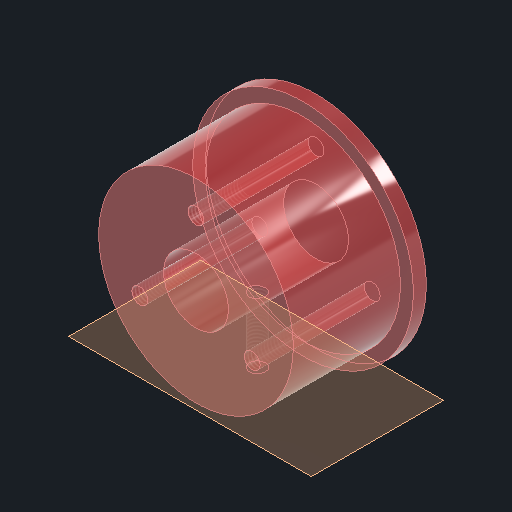
# Autodesk Inventor part: ReelMotorBearingShaft
Saved by Autodesk Inventor 2027 (Build 310192060, 192F)
## iProperties
Created: 2024-02-11
Part Number: ReelMotorBearingShaft
Material: Aluminum 6061
Document SubType Name: Modeling
Designer: Vinicius
Density: 2.7 g/cm^3
Appearance: Dark Red
Mass: 31.7586 g
Surface Area: 44.0893 cm^2
Volume: 11.7624 cm^3
Author: Vinicius
Autodesk Inventor part; units mm, degrees
ref_plane "YZ Plane" through (0, 0, 0) normal (1, 0, 0) x (0, 1, 0)
ref_plane "XY Plane" through (0, 0, 0) normal (0, 0, 1) x (1, 0, 0)
sketch "Sketch1" plane through (0, 0, 0) normal (0, 1, 0) x (-1, 0, 0)
  line L0 (0, 0) -> (0, 34.0434)
  line L1 (5, 0) -> (5, 18.5)
  line L2 (5, 18.5) -> (15, 18.5)
  line L3 (15, 18.5) -> (15, 2)
  line L4 (15, 2) -> (17, 2)
  line L5 (17, 2) -> (17, 0)
  line L6 (17, 0) -> (5, 0)
  dimension "d0" = 10
  dimension "d1" = 2
  dimension "d2" = 2
  dimension "d3" = 30
  dimension "d4" = 16.5
  constraints: 14 end point, 5 perpendicular, 2 vertical, 1 horizontal alignment
  measures "d0" diameter of L1 L0
  measures "d1" distance from line of L4.end L3
  measures "d2" distance of L4.end L5.end
  measures "d3" diameter of L3 L0
  measures "d4" distance of L2.end L3.end
revolve "Revolution1" add sketch "Sketch1" angle 360 about axis through (0, 0, 0) along (0, 0, 1)
sketch "Sketch2" plane through (0, 0, 18.5) normal (0, 0, 1) x (1, 0, 0)
  circle A0 centre (0, 0) radius 5 projected
  circle A1 centre (0, 0) radius 15 projected
  circle A2 centre (0, 0) radius 5 projected
  line L0 (0, 5) -> (0, 15)
  point P0 (0, 10)
  point P1 (0, 10)
  point P2 (-8.6603, -5)
  point P3 (8.6603, -5)
  dimension "d8" = 360
  constraints: 3 vertical alignment, 2 end point, 1 coincident, 1 midpoint, 1 vertical, 6 other
hole "Hole1" at (0, 10, 18.5) at (-8.6603, -5, 18.5) at (8.6603, -5, 18.5) direction (0, 0, -1) diameter 2.459 end through all thread size "M3x0.5" class "6H" standard "ISO Metric profile"
ref_plane "Work Plane2" through (0, -15, 10.25) normal (0, 1, 0) x (-1, 0, 0)
sketch "Sketch3" plane through (0, -15, 10.25) normal (0, 1, 0) x (-1, 0, 0)
  line L0 (17, -10.25) -> (-17, -10.25) projected
  point P0 (0, -10.25)
  point P1 (0, -1.25)
  point P2 (0, -10.25)
  dimension "d17" = 9
  constraints: 1 midpoint, 1 vertical alignment
  measures "d17" distance from line of L0 point (0, -1.25)
hole "Hole2" at (0, -15, 9) direction (0, 1, 0) diameter 2.459 depth 12 tip angle 118 thread size "M3x0.5" class "6H" standard "ISO Metric profile"
body "Solid1"
